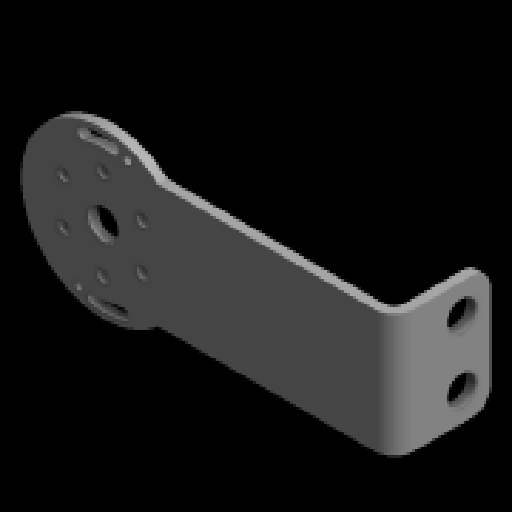
# Autodesk Inventor part: NeckPotentiometerBracket
Saved by Autodesk Inventor 2025.2 (Build 292293000, 293)
## iProperties
Created: 2025-09-15
Part Number: NeckPotentiometerBracket
Material: Generic
Document SubType Name: Sheet Metal
Designer: valer
Density: 1 g/cm^3
Sheet Metal Rule: Default_mm
Appearance: Default
Author: valer
Autodesk Inventor part; units mm, degrees
ref_plane "YZ Plane" through (0, 0, 0) normal (1, 0, 0) x (0, 1, 0)
ref_plane "XZ Plane" through (0, 0, 0) normal (0, 1, 0) x (-1, 0, 0)
ref_plane "XY Plane" through (0, 0, 0) normal (0, 0, 1) x (1, 0, 0)
sketch "Base" plane through (0, 0, 0) normal (0, 0, 1) x (1, 0, 0)
  circle A0 centre (0, 0) radius 3.125
  circle A1 centre (0, 0) radius 12.7
  line L0 (0, 12.7) -> (60, 12.7)
  line L1 (60, 12.7) -> (60, -12.7)
  line L2 (60, -12.7) -> (0, -12.7)
  dimension "d0" = 6.25
  dimension "d1" = 25.4
  dimension "d2" = 60
  measures "d0" diameter of A0
  measures "d1" diameter of A1
  measures "d2" distance of L0.start L0.end
extrude "Plate1" add sketch "Base" along normal blind 2
sketch "Sketch2" plane through (58, -12.7, 2) normal (1, 0, 0) x (0, 1, 0)
  line L0 (25.4, 0) -> (0, 0)
  line L1 (0, 0) -> (0, -20)
  line L2 (0, -20) -> (25.4, -20)
  line L3 (25.4, -20) -> (25.4, 0)
  constraints: 6 end point, 1 horizontal, 1 perpendicular, 1 vertical
edge flange "MountFeature" height 20 angle 90 thickness 2 bend radius 2 thickness toward (1, 0, 0) relief tear relief width 2 relief depth 1 edges at (60, 0, 0) wall of the first edge with corners at (58, 12.7, 2) (58, -12.7, 2) (58, -12.7, -18) (58, 12.7, -18)
bend "Bend1"
corner "Corner1"
fillet "MountFilletsFeature" radius 4 2 edges at (59, -12.7, -18) (59, 12.7, -18)
sketch "HubMountHoles" plane through (0, 0, 2) normal (0, 0, 1) x (1, 0, 0)
  circle A0 centre (0, 9.35) radius 1.25 projected
  circle A1 centre (8.0973, 4.675) radius 1.25 projected
  circle A2 centre (8.0973, -4.675) radius 1.25 projected
  circle A3 centre (0, -9.35) radius 1.25 projected
  circle A4 centre (-8.0973, -4.675) radius 1.25 projected
  circle A5 centre (-8.0973, 4.675) radius 1.25 projected
  point P0 (0, 0)
extrude "HubMountHolesFeature" cut sketch "HubMountHoles" against normal blind 2
sketch "PotMountHoles" plane through (0, 0, 2) normal (0, 0, 1) x (1, 0, 0)
  arc A0 (2.191, 15.5897) -> (-4.4715, 15.0972) centre (0.0082, -0.192) ccw
  arc A1 (-4.4715, 15.0972) -> (-3.8455, 12.9843) centre (-4.1585, 14.0408) ccw
  arc A2 (1.887, 13.4273) -> (-3.8455, 12.9843) centre (0.0734, -0.4153) ccw
  arc A3 (1.887, 13.4273) -> (2.191, 15.5897) centre (2.0448, 14.5077) ccw
  circle A4 centre (5.0089, 13.7622) radius 0.75
  circle A5 centre (-5.0089, -13.7614) radius 0.75
  arc A6 (-1.8863, -13.4212) -> (-2.1909, -15.5889) centre (-2.0386, -14.505) ccw
  arc A7 (-1.8863, -13.4212) -> (3.8453, -12.9835) centre (-0.0533, 0.3202) ccw
  arc A8 (-2.1909, -15.5889) -> (4.5487, -15.0702) centre (-0.0101, 0.1221) ccw
  arc A9 (4.5487, -15.0702) -> (3.8453, -12.9835) centre (4.1564, -14.0405) ccw
  circle A10 centre (0, 0) radius 3.125
  circle A11 centre (0, 0) radius 17
  circle A12 centre (-8.0973, 4.675) radius 1.25
  circle A13 centre (0, 9.35) radius 1.25
  circle A14 centre (8.0973, 4.675) radius 1.25
  circle A15 centre (8.0973, -4.675) radius 1.25
  circle A16 centre (0, -9.35) radius 1.25
  circle A17 centre (-8.0973, -4.675) radius 1.25
  dimension "d17" = 34
  measures "d17" diameter of A11
sheet face with bend "PotMountHolesFeature" sketch "PotMountHoles" thickness 2 toward (0, 0, -1) bend radius 2
bend "Bend3"
sketch "Sketch5" plane through (60, -12.7, -2) normal (1, 0, 0) x (0, 0, -1)
  line L0 (0, 25.4) -> (12, 25.4) construction
  line L1 (12, 0) -> (0, 0) construction
  line L2 (10, 25.4) -> (10, 0) construction
  circle A0 centre (10, 19.4) radius 3
  circle A1 centre (10, 6) radius 3
  line L3 (16, 21.4) -> (16, 4) projected
  point P0 (-2, 12.7)
  dimension "d28" = 6
  dimension "d29" = 6
  dimension "d30" = 6
  dimension "d31" = 6
  dimension "d32" = 6
  constraints: 4 point on line, 2 centre point, 2 end point, 1 perpendicular
  measures "d28" diameter of A0
  measures "d29" diameter of A1
  measures "d30" distance between parallel lines of L3 L2
  measures "d31" distance from line of L0 A0.centre
  measures "d32" distance from line of L1 A1.centre
extrude "Cut2" cut sketch "Sketch5" against normal blind 2
equation "\"d15\" = Thickness"
equation "\"d33\" = Thickness"
equation "\"d3\" = Thickness"
equation "\"d4\" = BendReliefWidth"
equation "\"d5\" = BendReliefDepth"
equation "\"d6\" = MinimumRemnant"
equation "\"d7\" = TransitionRadius"
equation "\"d10\" = BendRadius"
equation "\"d11\" = CornerReliefSize"
equation "\"d12\" = GapSize"
equation "\"d13\" = JacobiRadiusSize"
equation "\"d23\" = BendRadius"
equation "\"d24\" = BendReliefWidth"
equation "\"d26\" = MinimumRemnant"
equation "\"d25\" = BendReliefDepth"
equation "\"d27\" = TransitionRadius"
equation "\"BendRadius\" = Thickness"
equation "\"BendReliefWidth\" = Thickness"
equation "\"BendReliefDepth\" = 0.5 * Thickness"
equation "\"CornerReliefSize\" = 4 * Thickness"
equation "\"MinimumRemnant\" = 2 * Thickness"
equation "\"TransitionRadius\" = BendRadius"
equation "\"JacobiRadiusSize\" = BendRadius"
equation "\"GapSize\" = Thickness"
equation "\"Thickness\" = 2"
body "Solid1"
